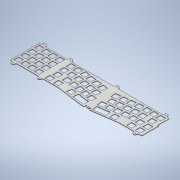
# Autodesk Inventor part: switch plate
Saved by Autodesk Inventor 2020 (Build 240168000, 168)
## iProperties
Created: 2019-02-21
Part Number: switch plate
Material: Generic
Document SubType Name: Modeling
Designer: Holt
Density: 1 g/cm^3
Appearance: Default
Author: Holt
Autodesk Inventor part; units mm, degrees
ref_plane "YZ Plane" through (0, 0, 0) normal (1, 0, 0) x (0, 1, 0)
ref_plane "XZ Plane" through (0, 0, 0) normal (0, 1, 0) x (-1, 0, 0)
ref_plane "XY Plane" through (0, 0, 0) normal (0, 0, 1) x (1, 0, 0)
sketch "Sketch1" plane through (0, 0, 0) normal (0, 0, 1) x (1, 0, 0)
  line L0 (224.769, 28.9898) -> (221.823, 29.4046)
  line L1 (221.823, 29.4046) -> (219.874, 15.5401)
  line L2 (219.874, 15.5401) -> (252.603, 10.9416)
  line L3 (252.603, 10.9416) -> (254.551, 24.8047)
  line L4 (254.551, 24.8047) -> (251.605, 25.2181)
  line L5 (251.605, 25.2181) -> (251.74, 26.1786)
  line L6 (251.74, 26.1786) -> (248.471, 26.6389)
  line L7 (248.471, 26.6389) -> (248.336, 25.6784)
  line L8 (248.336, 25.6784) -> (228.036, 28.5309)
  line L9 (228.036, 28.5309) -> (228.171, 29.4914)
  line L10 (228.171, 29.4914) -> (224.904, 29.9516)
  line L11 (224.904, 29.9516) -> (224.769, 28.9898)
  line L12 (198.651, 18.5236) -> (212.514, 16.5751)
  line L13 (212.514, 16.5751) -> (214.464, 30.4381)
  line L14 (214.464, 30.4381) -> (200.6, 32.3867)
  line L15 (200.6, 32.3867) -> (198.651, 18.5236)
  line L16 (319.1, 31.1021) -> (321.049, 17.2391)
  line L17 (321.049, 17.2391) -> (334.913, 19.1876)
  line L18 (334.913, 19.1876) -> (332.965, 33.052)
  line L19 (332.965, 33.052) -> (319.1, 31.1021)
  line L20 (136.826, 35.0848) -> (150.826, 35.0848)
  line L21 (150.826, 35.0848) -> (150.826, 21.0854)
  line L22 (150.826, 21.0854) -> (136.826, 21.0854)
  line L23 (136.826, 21.0854) -> (136.826, 35.0848)
  line L24 (160.638, 35.0848) -> (174.637, 35.0848)
  line L25 (174.637, 35.0848) -> (174.637, 21.0854)
  line L26 (174.637, 21.0854) -> (160.638, 21.0854)
  line L27 (160.638, 21.0854) -> (160.638, 35.0848)
  line L28 (363.615, 34.933) -> (377.617, 34.933)
  line L29 (377.617, 34.933) -> (377.617, 20.9336)
  line L30 (377.617, 20.9336) -> (363.615, 20.9336)
  line L31 (363.615, 20.9336) -> (363.615, 34.933)
  line L32 (387.427, 34.933) -> (401.426, 34.933)
  line L33 (401.426, 34.933) -> (401.426, 20.9336)
  line L34 (401.426, 20.9336) -> (387.427, 20.9336)
  line L35 (387.427, 20.9336) -> (387.427, 34.933)
  line L36 (241.39, 31.7541) -> (255.254, 29.8056)
  line L37 (255.254, 29.8056) -> (257.201, 43.6686)
  line L38 (257.201, 43.6686) -> (243.338, 45.6188)
  line L39 (243.338, 45.6188) -> (241.39, 31.7541)
  line L40 (271.646, 43.6699) -> (273.595, 29.8068)
  line L41 (273.595, 29.8068) -> (287.459, 31.7553)
  line L42 (287.459, 31.7553) -> (285.509, 45.6197)
  line L43 (285.509, 45.6197) -> (271.646, 43.6699)
  line L44 (222.526, 34.4055) -> (236.389, 32.4569)
  line L45 (236.389, 32.4569) -> (238.337, 46.3201)
  line L46 (238.337, 46.3201) -> (224.474, 48.2685)
  line L47 (224.474, 48.2685) -> (222.526, 34.4055)
  line L48 (290.51, 46.321) -> (292.459, 32.4581)
  line L49 (292.459, 32.4581) -> (306.323, 34.4066)
  line L50 (306.323, 34.4066) -> (304.375, 48.2712)
  line L51 (304.375, 48.2712) -> (290.51, 46.321)
  line L52 (203.66, 37.0568) -> (217.525, 35.1083)
  line L53 (217.525, 35.1083) -> (219.473, 48.9726)
  line L54 (219.473, 48.9726) -> (205.609, 50.9199)
  line L55 (205.609, 50.9199) -> (203.66, 37.0568)
  line L56 (309.376, 48.9739) -> (311.324, 35.1094)
  line L57 (311.324, 35.1094) -> (325.187, 37.0581)
  line L58 (325.187, 37.0581) -> (323.239, 50.9209)
  line L59 (323.239, 50.9209) -> (309.376, 48.9739)
  line L60 (184.796, 39.7083) -> (198.659, 37.7596)
  line L61 (198.659, 37.7596) -> (200.609, 51.6227)
  line L62 (200.609, 51.6227) -> (186.745, 53.5711)
  line L63 (186.745, 53.5711) -> (184.796, 39.7083)
  line L64 (328.239, 51.624) -> (330.188, 37.7609)
  line L65 (330.188, 37.7609) -> (344.051, 39.7093)
  line L66 (344.051, 39.7093) -> (342.104, 53.5724)
  line L67 (342.104, 53.5724) -> (328.239, 51.624)
  line L68 (139.493, 54.325) -> (153.493, 54.325)
  line L69 (153.493, 54.325) -> (153.493, 40.3243)
  line L70 (153.493, 40.3243) -> (139.493, 40.3243)
  line L71 (139.493, 40.3243) -> (139.493, 54.325)
  line L72 (165.687, 54.325) -> (179.687, 54.325)
  line L73 (179.687, 54.325) -> (179.687, 40.3243)
  line L74 (179.687, 40.3243) -> (165.687, 40.3243)
  line L75 (165.687, 40.3243) -> (165.687, 54.325)
  line L76 (349.042, 54.1732) -> (363.043, 54.1732)
  line L77 (363.043, 54.1732) -> (363.043, 40.1725)
  line L78 (363.043, 40.1725) -> (349.042, 40.1725)
  line L79 (349.042, 40.1725) -> (349.042, 54.1732)
  line L80 (368.092, 54.1732) -> (382.093, 54.1732)
  line L81 (382.093, 54.1732) -> (382.093, 40.1725)
  line L82 (382.093, 40.1725) -> (368.092, 40.1725)
  line L83 (368.092, 40.1725) -> (368.092, 54.1732)
  line L84 (389.523, 54.1732) -> (403.525, 54.1732)
  line L85 (403.525, 54.1732) -> (403.525, 40.1725)
  line L86 (403.525, 40.1725) -> (389.523, 40.1725)
  line L87 (389.523, 40.1725) -> (389.523, 54.1732)
  line L88 (234.608, 51.9437) -> (248.473, 49.9967)
  line L89 (248.473, 49.9967) -> (250.421, 63.8598)
  line L90 (250.421, 63.8598) -> (236.558, 65.8082)
  line L91 (236.558, 65.8082) -> (234.608, 51.9437)
  line L92 (278.426, 63.8608) -> (280.376, 49.9977)
  line L93 (280.376, 49.9977) -> (294.239, 51.945)
  line L94 (294.239, 51.945) -> (292.291, 65.8095)
  line L95 (292.291, 65.8095) -> (278.426, 63.8608)
  line L96 (215.744, 54.5952) -> (229.607, 52.6464)
  line L97 (229.607, 52.6464) -> (231.557, 66.511)
  line L98 (231.557, 66.511) -> (217.693, 68.4597)
  line L99 (217.693, 68.4597) -> (215.744, 54.5952)
  line L100 (297.292, 66.5123) -> (299.24, 52.6477)
  line L101 (299.24, 52.6477) -> (313.103, 54.5961)
  line L102 (313.103, 54.5961) -> (311.156, 68.4607)
  line L103 (311.156, 68.4607) -> (297.292, 66.5123)
  line L104 (196.88, 57.2463) -> (210.743, 55.2979)
  line L105 (210.743, 55.2979) -> (212.692, 69.1624)
  line L106 (212.692, 69.1624) -> (198.827, 71.1094)
  line L107 (198.827, 71.1094) -> (196.88, 57.2463)
  line L108 (316.157, 69.1634) -> (318.105, 55.2992)
  line L109 (318.105, 55.2992) -> (331.969, 57.249)
  line L110 (331.969, 57.249) -> (330.02, 71.1121)
  line L111 (330.02, 71.1121) -> (316.157, 69.1634)
  line L112 (178.015, 59.8978) -> (191.879, 57.9494)
  line L113 (191.879, 57.9494) -> (193.827, 71.8136)
  line L114 (193.827, 71.8136) -> (179.964, 73.7609)
  line L115 (179.964, 73.7609) -> (178.015, 59.8978)
  line L116 (335.021, 71.8149) -> (336.97, 57.9503)
  line L117 (336.97, 57.9503) -> (350.832, 59.8991)
  line L118 (350.832, 59.8991) -> (348.885, 73.7633)
  line L119 (348.885, 73.7633) -> (335.021, 71.8149)
  line L120 (137.682, 73.5665) -> (151.684, 73.5665)
  line L121 (151.684, 73.5665) -> (151.684, 59.5644)
  line L122 (151.684, 59.5644) -> (137.682, 59.5644)
  line L123 (137.682, 59.5644) -> (137.682, 73.5665)
  line L124 (159.019, 73.5665) -> (173.018, 73.5665)
  line L125 (173.018, 73.5665) -> (173.018, 59.5644)
  line L126 (173.018, 59.5644) -> (159.019, 59.5644)
  line L127 (159.019, 59.5644) -> (159.019, 73.5665)
  line L128 (355.9, 73.4147) -> (369.901, 73.4147)
  line L129 (369.901, 73.4147) -> (369.901, 59.4126)
  line L130 (369.901, 59.4126) -> (355.9, 59.4126)
  line L131 (355.9, 59.4126) -> (355.9, 73.4147)
  line L132 (382.093, 73.4147) -> (396.095, 73.4147)
  line L133 (396.095, 73.4147) -> (396.095, 59.4126)
  line L134 (396.095, 59.4126) -> (382.093, 59.4126)
  line L135 (382.093, 59.4126) -> (382.093, 73.4147)
  line L136 (271.059, 82.062) -> (273.008, 68.1989)
  line L137 (273.008, 68.1989) -> (286.872, 70.1473)
  line L138 (286.872, 70.1473) -> (284.924, 84.0118)
  line L139 (284.924, 84.0118) -> (271.059, 82.062)
  line L140 (232.5558, 71.4724) -> (246.4211, 69.534)
  line L141 (246.4211, 69.534) -> (248.36, 83.3998)
  line L142 (248.36, 83.3998) -> (234.4947, 85.3381)
  line L143 (234.4947, 85.3381) -> (232.5558, 71.4724)
  line L144 (289.925, 84.7135) -> (291.873, 70.8504)
  line L145 (291.873, 70.8504) -> (305.736, 72.7988)
  line L146 (305.736, 72.7988) -> (303.788, 86.6619)
  line L147 (303.788, 86.6619) -> (289.925, 84.7135)
  line L148 (213.6831, 74.1236) -> (227.5465, 72.1776)
  line L149 (227.5465, 72.1776) -> (229.4921, 86.0411)
  line L150 (229.4921, 86.0411) -> (215.6277, 87.9871)
  line L151 (215.6277, 87.9871) -> (213.6831, 74.1236)
  line L152 (308.7877, 87.3634) -> (310.7292, 73.498)
  line L153 (310.7292, 73.498) -> (324.5931, 75.4388)
  line L154 (324.5931, 75.4388) -> (322.6526, 89.3043)
  line L155 (322.6526, 89.3043) -> (308.7877, 87.3634)
  line L156 (194.8151, 76.7745) -> (208.6802, 74.8256)
  line L157 (208.6802, 74.8256) -> (210.6263, 88.6898)
  line L158 (210.6263, 88.6898) -> (196.7632, 90.6378)
  line L159 (196.7632, 90.6378) -> (194.8151, 76.7745)
  line L160 (327.6601, 90.017) -> (329.6334, 76.1573)
  line L161 (329.6334, 76.1573) -> (343.4929, 78.13)
  line L162 (343.4929, 78.13) -> (341.5207, 91.9896)
  line L163 (341.5207, 91.9896) -> (327.6601, 90.017)
  line L164 (175.949, 79.4247) -> (189.814, 77.4774)
  line L165 (189.814, 77.4774) -> (191.762, 91.3405)
  line L166 (191.762, 91.3405) -> (177.899, 93.2889)
  line L167 (177.899, 93.2889) -> (175.949, 79.4247)
  line L168 (367.52, 92.6549) -> (367.52, 78.6542)
  line L169 (367.52, 78.6542) -> (381.52, 78.6542)
  line L170 (381.52, 78.6542) -> (381.52, 92.6549)
  line L171 (381.52, 92.6549) -> (367.52, 92.6549)
  line L172 (400.572, 78.6542) -> (400.572, 92.6549)
  line L173 (400.572, 92.6549) -> (386.572, 92.6549)
  line L174 (386.572, 92.6549) -> (386.572, 78.6542)
  line L175 (386.572, 78.6542) -> (400.572, 78.6542)
  line L176 (137.874, 92.8067) -> (151.874, 92.8067)
  line L177 (151.874, 92.8067) -> (151.874, 78.8046)
  line L178 (151.874, 78.8046) -> (137.874, 78.8046)
  line L179 (137.874, 78.8046) -> (137.874, 92.8067)
  line L180 (156.924, 92.8067) -> (170.924, 92.8067)
  line L181 (170.924, 92.8067) -> (170.924, 78.8046)
  line L182 (170.924, 78.8046) -> (156.924, 78.8046)
  line L183 (156.924, 78.8046) -> (156.924, 92.8067)
  line L184 (348.47, 92.6549) -> (362.472, 92.6549)
  line L185 (362.472, 92.6549) -> (362.472, 78.6528)
  line L186 (362.472, 78.6528) -> (348.47, 78.6528)
  line L187 (348.47, 78.6528) -> (348.47, 92.6549)
  line L188 (282.8681, 26.0103) -> (303.1679, 28.8637)
  line L189 (303.1679, 28.8637) -> (303.033, 29.8243)
  line L190 (303.033, 29.8243) -> (306.3022, 30.2828)
  line L191 (306.3022, 30.2828) -> (306.4372, 29.3223)
  line L192 (306.4372, 29.3223) -> (309.383, 29.737)
  line L193 (309.383, 29.737) -> (311.3317, 15.874)
  line L194 (311.3317, 15.874) -> (278.603, 11.273)
  line L195 (278.603, 11.273) -> (276.6549, 25.1376)
  line L196 (276.6549, 25.1376) -> (279.6011, 25.5509)
  line L197 (279.6011, 25.5509) -> (279.4658, 26.5127)
  line L198 (279.4658, 26.5127) -> (282.7331, 26.9708)
  line L199 (282.7331, 26.9708) -> (282.8681, 26.0103)
  line L200 (106.443, 92.8067) -> (120.443, 92.8067)
  line L201 (120.443, 92.8067) -> (120.443, 78.8067)
  line L202 (120.443, 78.8067) -> (106.443, 78.8067)
  line L203 (106.443, 78.8067) -> (106.443, 92.8067)
  line L204 (101.393, 78.8067) -> (101.393, 92.8067)
  line L205 (101.393, 92.8067) -> (87.393, 92.8067)
  line L206 (87.393, 92.8067) -> (87.393, 78.8067)
  line L207 (87.393, 78.8067) -> (101.393, 78.8067)
  line L208 (82.343, 78.8067) -> (82.343, 92.8067)
  line L209 (82.343, 92.8067) -> (68.343, 92.8067)
  line L210 (68.343, 92.8067) -> (68.343, 78.8067)
  line L211 (68.343, 78.8067) -> (82.343, 78.8067)
  line L212 (63.293, 78.8067) -> (63.293, 92.8067)
  line L213 (63.293, 92.8067) -> (49.293, 92.8067)
  line L214 (49.293, 92.8067) -> (49.293, 78.8067)
  line L215 (49.293, 78.8067) -> (63.293, 78.8067)
  line L216 (120.443, 59.7567) -> (120.443, 73.7567)
  line L217 (120.443, 73.7567) -> (106.443, 73.7567)
  line L218 (106.443, 73.7567) -> (106.443, 59.7567)
  line L219 (106.443, 59.7567) -> (120.443, 59.7567)
  line L220 (101.393, 59.7567) -> (101.393, 73.7567)
  line L221 (101.393, 73.7567) -> (87.393, 73.7567)
  line L222 (87.393, 73.7567) -> (87.393, 59.7567)
  line L223 (87.393, 59.7567) -> (101.393, 59.7567)
  line L224 (82.343, 59.7567) -> (82.343, 73.7567)
  line L225 (82.343, 73.7567) -> (68.343, 73.7567)
  line L226 (68.343, 73.7567) -> (68.343, 59.7567)
  line L227 (68.343, 59.7567) -> (82.343, 59.7567)
  line L228 (63.293, 59.7567) -> (63.293, 73.7567)
  line L229 (63.293, 73.7567) -> (49.293, 73.7567)
  line L230 (49.293, 73.7567) -> (49.293, 59.7567)
  line L231 (49.293, 59.7567) -> (63.293, 59.7567)
  line L232 (120.443, 40.7067) -> (120.443, 54.7067)
  line L233 (120.443, 54.7067) -> (106.443, 54.7067)
  line L234 (106.443, 54.7067) -> (106.443, 40.7067)
  line L235 (106.443, 40.7067) -> (120.443, 40.7067)
  line L236 (101.393, 40.7067) -> (101.393, 54.7067)
  line L237 (101.393, 54.7067) -> (87.393, 54.7067)
  line L238 (87.393, 54.7067) -> (87.393, 40.7067)
  line L239 (87.393, 40.7067) -> (101.393, 40.7067)
  line L240 (82.343, 40.7067) -> (82.343, 54.7067)
  line L241 (82.343, 54.7067) -> (68.343, 54.7067)
  line L242 (68.343, 54.7067) -> (68.343, 40.7067)
  line L243 (68.343, 40.7067) -> (82.343, 40.7067)
  line L244 (63.293, 40.7067) -> (63.293, 54.7067)
  line L245 (63.293, 54.7067) -> (49.293, 54.7067)
  line L246 (49.293, 54.7067) -> (49.293, 40.7067)
  line L247 (49.293, 40.7067) -> (63.293, 40.7067)
  line L248 (120.443, 21.6567) -> (120.443, 35.6567)
  line L249 (120.443, 35.6567) -> (106.443, 35.6567)
  line L250 (106.443, 35.6567) -> (106.443, 21.6567)
  line L251 (106.443, 21.6567) -> (120.443, 21.6567)
  line L252 (101.393, 21.6567) -> (101.393, 35.6567)
  line L253 (101.393, 35.6567) -> (87.393, 35.6567)
  line L254 (87.393, 35.6567) -> (87.393, 21.6567)
  line L255 (87.393, 21.6567) -> (101.393, 21.6567)
  line L256 (82.343, 21.6567) -> (82.343, 35.6567)
  line L257 (82.343, 35.6567) -> (68.343, 35.6567)
  line L258 (68.343, 35.6567) -> (68.343, 21.6567)
  line L259 (68.343, 21.6567) -> (82.343, 21.6567)
  line L260 (63.293, 21.6567) -> (63.293, 35.6567)
  line L261 (63.293, 35.6567) -> (49.293, 35.6567)
  line L262 (49.293, 35.6567) -> (49.293, 21.6567)
  line L263 (49.293, 21.6567) -> (63.293, 21.6567)
  line L264 (172.4586, 79.9171) -> (172.4584, 79.9157)
  line L265 (150.826, 17.0854) -> (136.826, 17.0854)
  line L266 (174.637, 17.0854) -> (160.638, 17.0854)
  line L267 (198.0943, 14.5625) -> (211.9573, 12.614)
  line L268 (219.3175, 11.579) -> (252.0465, 6.9805)
  line L269 (311.8885, 11.9129) -> (276.8022, 6.9805)
  line L270 (321.6057, 13.278) -> (347.6159, 16.9336)
  line L271 (407.525, 54.1732) -> (407.525, 40.1725)
  line L272 (136.826, 17.0854) -> (123.5393, 17.0854)
  line L273 (150.826, 17.0854) -> (160.638, 17.0854)
  line L274 (174.637, 17.0854) -> (180.1448, 17.0854)
  line L275 (198.0943, 14.5625) -> (180.1448, 17.0854)
  line L276 (211.9573, 12.614) -> (219.3175, 11.579)
  line L277 (311.8885, 11.9129) -> (321.6057, 13.278)
  line L278 (407.525, 54.1732) -> (407.525, 56.6982)
  line L279 (407.525, 40.1725) -> (407.525, 37.6475)
  line L280 (407.525, 56.6982) -> (407.525, 96.598)
  line L281 (407.525, 37.6475) -> (407.525, 16.9336)
  line L282 (181.6096, 96.8067) -> (407.525, 96.598)
  line L283 (45.293, 96.8067) -> (181.6096, 96.8067)
  line L284 (347.6159, 16.9336) -> (407.525, 16.9336)
  line L285 (45.293, 96.8067) -> (45.293, 17.6567)
  line L286 (123.5393, 17.0854) -> (45.293, 17.0854)
  line L287 (45.293, 17.0854) -> (45.293, 17.6567)
  line L288 (252.0465, 6.9805) -> (276.8022, 6.9805)
  point P0 (0, 0)
  dimension "d0" = 14
  dimension "d63" = 16.383
  dimension "d64" = 5.05
  dimension "d65" = 5.05
  dimension "d66" = 5.05
  dimension "d67" = 14
  dimension "d73" = 4
  dimension "d74" = 4
  dimension "d75" = 4
  dimension "d76" = 4
  dimension "d77" = 4
  dimension "d78" = 4
  dimension "d81" = 4
  dimension "d84" = 5.2381
  constraints: 578 end point, 7 parallel, 5 horizontal, 4 vertical, 2 collinear, 2 perpendicular
  measures "d0" distance of L208.end L209.end
  measures "d63" distance between parallel lines of L23 L248
  measures "d64" distance between parallel lines of L252 L250
  measures "d65" distance between parallel lines of L256 L254
  measures "d66" distance between parallel lines of L260 L258
  measures "d67" distance of L260.end L261.end
  measures "d73" distance between parallel lines of L22 L265
  measures "d74" distance between parallel lines of L26 L266
  measures "d75" distance between parallel lines of L12 L267
  measures "d76" distance between parallel lines of L2 L268
  measures "d77" distance between parallel lines of L194 L269
  measures "d78" distance between parallel lines of L17 L270
  measures "d81" distance between parallel lines of L85 L271
  measures "d84" distance between parallel lines of L120 L178
extrude "Extrusion1" add sketch "Sketch1" along normal blind 1.5
move faces "Move1" translate (2, 0, 0) faces at (407.525, 23.8382, 1) (407.525, 38.4892, 0.5) (407.525, 44.8394, 0.5) (407.525, 55.0149, 0.5) (407.525, 69.9981, 0.5)
sketch "Sketch2" plane through (0, 0, 1.5) normal (0, 0, 1) x (1, 0, 0)
  line L0 (49.293, 92.8067) -> (63.293, 92.8067) projected
  line L1 (63.293, 21.6567) -> (49.293, 21.6567) projected
  line L2 (401.426, 20.9336) -> (387.427, 20.9336) projected
  line L3 (386.572, 92.6549) -> (400.572, 92.6549) projected
  line L4 (137.874, 92.8067) -> (151.874, 92.8067) projected
  line L5 (120.443, 92.8067) -> (137.874, 92.8067)
  circle A0 centre (56.293, 99.3067) radius 1.1
  line L6 (181.6096, 96.8067) -> (45.293, 96.8067) projected
  circle A1 centre (56.293, 14.5854) radius 1.1
  line L7 (45.293, 17.0854) -> (180.1448, 17.0854) projected
  circle A2 centre (393.5697, 99.1109) radius 1.1
  line L8 (409.525, 96.5962) -> (181.6096, 96.8067) projected
  circle A3 centre (394.4265, 14.4336) radius 1.1
  line L9 (347.6159, 16.9336) -> (409.525, 16.9336) projected
  arc A4 (389.3265, 14.4336) -> (399.5265, 14.4336) centre (394.4265, 14.4336) ccw
  line L10 (389.3265, 16.9336) -> (389.3265, 14.4336)
  line L11 (399.5265, 16.9336) -> (399.5265, 14.4336)
  line L12 (252.0465, 6.9805) -> (276.8022, 6.9805) projected
  line L13 (252.0465, 6.9805) -> (276.8022, 6.9805) projected
  circle A5 centre (258.7815, 99.2354) radius 1.1
  arc A6 (263.8815, 99.2354) -> (253.6815, 99.2354) centre (258.7815, 99.2354) ccw
  line L14 (409.525, 96.5962) -> (181.6096, 96.8067) projected
  line L15 (253.6815, 96.7401) -> (253.6815, 99.2354)
  line L16 (263.8815, 96.7307) -> (263.8815, 99.2354)
  circle A7 centre (129.1585, 99.3067) radius 1.1
  arc A8 (134.2585, 99.3067) -> (124.0585, 99.3067) centre (129.1585, 99.3067) ccw
  line L17 (181.6096, 96.8067) -> (45.293, 96.8067) projected
  line L18 (124.0585, 96.8067) -> (124.0585, 99.3067)
  line L19 (134.2585, 96.8067) -> (134.2585, 99.3067)
  circle A9 centre (129.1585, 14.5854) radius 1.1
  arc A10 (124.0585, 14.5854) -> (134.2585, 14.5854) centre (129.1585, 14.5854) ccw
  line L20 (124.0585, 17.0854) -> (124.0585, 14.5854)
  line L21 (134.2585, 17.0854) -> (134.2585, 14.5854)
  arc A11 (61.393, 99.3067) -> (51.193, 99.3067) centre (56.293, 99.3067) ccw
  line L22 (51.193, 96.8067) -> (51.193, 99.3067)
  line L23 (61.393, 96.8067) -> (61.393, 99.3067)
  arc A12 (398.6697, 99.1109) -> (388.4697, 99.1109) centre (393.5697, 99.1109) ccw
  line L24 (388.4697, 96.6156) -> (388.4697, 99.1109)
  line L25 (398.6697, 96.6062) -> (398.6697, 99.1109)
  arc A13 (51.193, 14.5854) -> (61.393, 14.5854) centre (56.293, 14.5854) ccw
  line L26 (51.193, 17.0854) -> (51.193, 14.5854)
  line L27 (61.393, 17.0854) -> (61.393, 14.5854)
  point P0 (0, 0)
  point P1 (50.693, 96.8067)
  point P2 (61.893, 96.8067)
  point P3 (61.893, 17.0854)
  point P4 (50.693, 17.0854)
  point P5 (387.9697, 96.6161)
  point P6 (399.1697, 96.6057)
  point P7 (263.8815, 96.7307)
  dimension "d94" = 2.2
  dimension "d96" = 2.5
  dimension "d97" = 2.2
  dimension "d98" = 2.5
  dimension "d100" = 2.2
  dimension "d101" = 2.5
  dimension "d103" = 2.2
  dimension "d104" = 2.5
  dimension "d105" = 4
  dimension "d109" = 2.2
  dimension "d110" = 2.5
  dimension "d111" = 4
  dimension "d112" = 2.2
  dimension "d113" = 2.5
  dimension "d114" = 4
  dimension "d115" = 2.2
  dimension "d116" = 2.5
  dimension "d117" = 4
  dimension "d138" = 4
  dimension "d139" = 4
  dimension "d140" = 4
  constraints: 30 end point, 20 point on line, 14 centre point, 14 point on circle, 14 tangent, 1 horizontal
  measures "d94" diameter of A0
  measures "d96" distance from line of L6 A0.centre
  measures "d97" diameter of A1
  measures "d98" distance from line of L7 A1.centre
  measures "d100" diameter of A2
  measures "d101" distance from line of L8 A2.centre
  measures "d103" diameter of A3
  measures "d104" distance from line of L9 A3.centre
  measures "d105" radial gap between concentric circles of A3 A4
  measures "d109" diameter of A5
  measures "d110" distance from line of L8 A5.centre
  measures "d111" radial gap between concentric circles of A5 A6
  measures "d112" diameter of A7
  measures "d113" distance from line of L6 A7.centre
  measures "d114" radial gap between concentric circles of A7 A8
  measures "d115" diameter of A9
  measures "d116" distance from line of L7 A9.centre
  measures "d117" radial gap between concentric circles of A9 A10
  measures "d138" radial gap between concentric circles of A0 A11
  measures "d139" radial gap between concentric circles of A2 A12
  measures "d140" radial gap between concentric circles of A1 A13
extrude "Extrusion3" add sketch "Sketch2" against normal blind 1.5
sketch "Sketch3" plane through (0, 0, 1.5) normal (0, 0, 1) x (1, 0, 0)
  circle A0 centre (266.615, 12.9805) radius 1.1
  line L0 (252.0465, 6.9805) -> (276.8022, 6.9805) projected
  line L1 (363.615, 20.9336) -> (363.615, 34.933) projected
  circle A1 centre (266.615, 12.9805) radius 5.1
  line L2 (271.715, 12.9805) -> (273.715, 12.9805)
  line L3 (273.715, 12.9805) -> (273.715, 6.6426)
  line L4 (273.715, 6.6426) -> (261.0474, 6.6426)
  line L5 (261.515, 12.9805) -> (259.515, 12.9805)
  line L6 (259.515, 12.9805) -> (259.515, 6.6426)
  line L7 (259.515, 6.6426) -> (261.0474, 6.6426)
  point P0 (0, 0)
  point P1 (259.515, 6.9805)
  point P2 (273.715, 6.9805)
  dimension "d123" = 2.2
  dimension "d124" = 6
  dimension "d125" = 97
  dimension "d126" = 4
  dimension "d127" = 2
  dimension "d128" = 2
  constraints: 12 end point, 3 perpendicular, 2 centre point, 2 horizontal, 2 point on circle, 1 vertical
  measures "d123" diameter of A0
  measures "d124" distance from line of A0.centre L0
  measures "d125" distance from line of L1 A0.centre
  measures "d126" radial gap between concentric circles of A0 A1
  measures "d127" distance of L2.start L2.end
  measures "d128" distance of L5.start L5.end
extrude "Extrusion4" cut sketch "Sketch3" against normal blind 1.5 contours A0 | L6 L5 A1 L2 L3 L0
fillet "Fillet2" radius 2 20 edges at (124.0585, 17.0854, 0.75) (134.2585, 17.0854, 0.75) (124.0585, 96.8067, 0.75) (134.2585, 96.8067, 0.75) (253.6815, 96.7401, 0.75) (263.8815, 96.7307, 0.75) (399.5265, 16.9336, 0.75) (389.3265, 16.9336, 0.75) (259.515, 6.9805, 0.75) (273.715, 6.9805, 0.75) (409.525, 16.9336, 0.75) (409.525, 96.5962, 0.75) (45.293, 96.8067, 0.75) (45.293, 17.0854, 0.75) (61.393, 96.8067, 0.75) (51.193, 96.8067, 0.75) (51.193, 17.0854, 0.75) (61.393, 17.0854, 0.75) (398.6697, 96.6062, 0.75) (388.4697, 96.6156, 0.75)
sketch "Sketch4" plane through (0, 0, 1.5) normal (0, 0, 1) x (1, 0, 0)
  line L0 (407.5268, 96.598) -> (181.6096, 96.8067) projected
  line L1 (406.371, 64.3467) -> (409.525, 64.3467)
  line L2 (409.525, 18.9336) -> (409.525, 94.598) projected
  arc A0 (409.525, 94.598) -> (407.5268, 96.598) centre (407.525, 94.598) ccw projected
  line L3 (406.371, 64.3467) -> (406.371, 96.5991)
  point P0 (0, 0)
  point P1 (294.5682, 96.7024)
  point P2 (401.1679, 96.6039)
  constraints: 4 end point, 2 point on line, 1 horizontal, 1 midpoint, 1 perpendicular
extrude "Extrusion5" cut sketch "Sketch4" against normal blind 1.5
sketch "Sketch5" plane through (0, 0, 1.5) normal (0, 0, 1) x (1, 0, 0)
  line L0 (263.0025, 9.3805) -> (270.2275, 9.3805)
  circle A0 centre (266.615, 12.9805) radius 1.1 projected
  arc A1 (261.515, 12.9805) -> (271.715, 12.9805) centre (266.615, 12.9805) ccw projected
  point P0 (0, 0)
  dimension "d141" = 2.5
  constraints: 2 end point, 2 point on circle, 1 horizontal
  measures "d141" distance edge to line of A0 L0
extrude "Extrusion6" cut sketch "Sketch5" against normal blind 10 contours L0 A1
fillet "Fillet3" radius 2 2 edges at (263.0025, 9.3805, 0.75) (270.2275, 9.3805, 0.75)
body "Solid1"
